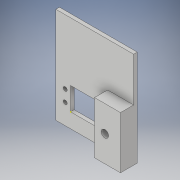
# Autodesk Inventor part: ClawServoHolder
Saved by Autodesk Inventor 2017 (Build 210142000, 142)
## iProperties
Created: 2017-09-23
Part Number: ClawServoHolder
Material: Generic
Document SubType Name: Modeling
Designer: User
Density: 1 g/cm^3
Appearance: Default
Author: User
Autodesk Inventor part; units mm, degrees
ref_plane "YZ Plane" through (0, 0, 0) normal (1, 0, 0) x (0, 1, 0)
ref_plane "XZ Plane" through (0, 0, 0) normal (0, 1, 0) x (-1, 0, 0)
ref_plane "XY Plane" through (0, 0, 0) normal (0, 0, 1) x (1, 0, 0)
sketch "Sketch1" plane through (0, 0, 0) normal (0, 0, 1) x (1, 0, 0)
  line L0 (0, 0) -> (38.8112, 0)
  line L1 (38.8112, 0) -> (38.8112, 19.812)
  line L2 (38.8112, 19.812) -> (0, 19.812)
  line L3 (0, 19.812) -> (0, 0)
  line L4 (-12.7, -12.7) -> (-12.7, 32.512)
  line L5 (-12.7, 32.512) -> (51.5112, 32.512)
  line L6 (51.5112, 32.512) -> (51.5112, -12.7)
  line L7 (-12.7, -12.7) -> (51.5112, -12.7)
  dimension "d0" = 38.8112
  dimension "d1" = 19.812
  constraints: 16 end point, 3 perpendicular, 2 horizontal, 2 parallel
  measures "d0" distance of L2.end L1.end
  measures "d1" distance of L1.end L0.end
extrude "Extrusion1" add sketch "Sketch1" along normal blind 3.175
sketch "Sketch2" plane through (0, 0, 3.175) normal (0, 0, 1) x (1, 0, 0)
  line L0 (0, 19.812) -> (0, 0) projected
  circle A0 centre (-4.5974, 4.9022) radius 1.0541
  line L1 (38.8112, 19.812) -> (38.8112, 0) projected
  circle A1 centre (43.4086, 4.9022) radius 1.0541
  circle A2 centre (43.4086, 14.9098) radius 1.0541
  circle A3 centre (-4.5974, 14.9098) radius 1.0541
  circle A4 centre (-4.5974, 4.9022) radius 1.7145
  circle A5 centre (-4.5974, 14.9098) radius 1.7145
  circle A6 centre (43.4086, 14.9098) radius 1.7145
  circle A7 centre (43.4086, 4.9022) radius 1.7145
  dimension "d10" = 2.1082
  dimension "d15" = 3.429
  dimension "d16" = 3.429
  dimension "d17" = 3.429
  dimension "d18" = 3.429
  dimension "d46" = 48.006
  dimension "d47" = 48.006
  constraints: 8 centre point, 5 coincident
  measures "d10" diameter of A0
  measures "d15" diameter of A4
  measures "d16" diameter of A5
  measures "d17" diameter of A6
  measures "d18" diameter of A7
  measures "d46" distance of A2.centre A3.centre
  measures "d47" distance of A1.centre A0.centre
extrude "Extrusion2" cut sketch "Sketch2" against normal blind 3.175 contours A0 | A1 | A2 | A3 | A4 | A5 | A6 | A7
sketch "Sketch3" plane through (51.5112, -12.7, 0) normal (1, 0, 0) x (0, 0, -1)
  line L0 (0, 0) -> (-3.175, 0) projected
  line L1 (-3.175, 0) -> (-3.175, 45.212) projected
  line L2 (0, 0) -> (-3.175, 0)
  line L3 (-3.175, 0) -> (-3.175, 45.212)
  line L4 (-3.175, 45.212) -> (0, 45.212)
  line L5 (0, 45.212) -> (0, 0)
  point P0 (0, 12.7)
  constraints: 8 end point, 2 parallel, 1 horizontal, 1 perpendicular
extrude "Extrusion3" add sketch "Sketch3" along normal blind 3.175
sketch "Sketch4" plane through (0, 0, 3.175) normal (0, 0, 1) x (1, 0, 0)
  line L0 (54.6862, 32.512) -> (54.6862, -12.7) projected
  line L1 (54.6862, 32.512) -> (51.5112, 32.512)
  line L2 (-12.7, 32.512) -> (54.6862, 32.512) projected
  line L3 (51.5112, 32.512) -> (51.2299, -12.7)
  line L4 (-12.7, -12.7) -> (54.6862, -12.7) projected
  line L5 (54.6862, -12.7) -> (51.2299, -12.7)
  point P0 (0, 0)
  dimension "d21" = 3.175
  constraints: 6 end point, 2 point on line, 1 collinear
  measures "d21" distance of L0.start L1.end
extrude "Extrusion4" add sketch "Sketch4" along normal blind 8.2296
sketch "Sketch8" plane through (0, 0, 3.175) normal (0, 0, 1) x (1, 0, 0)
  line L0 (51.2299, -12.7) -> (32.1799, -12.7)
  line L1 (-12.7, -12.7) -> (51.2299, -12.7) projected
  line L2 (38.8112, 0) -> (0, 0) projected
  line L3 (32.1799, -12.7) -> (32.1799, 32.512)
  line L4 (-12.7, 32.512) -> (51.5112, 32.512) projected
  line L5 (32.1799, 32.512) -> (51.5112, 32.512)
  line L6 (51.2299, -12.7) -> (51.5112, 32.512) projected
  line L7 (51.5112, 32.512) -> (51.2299, -12.7)
  dimension "d33" = 19.05
  dimension "d36" = 45.212
  constraints: 8 end point, 2 collinear, 2 point on line
  measures "d33" distance of L0.start L0.end
  measures "d36" distance of L0.end L3.end
extrude "Extrusion7" add sketch "Sketch8" along normal blind 8.2296
sketch "Sketch9" plane through (0, 0, 11.4046) normal (0, 0, 1) x (1, 0, 0)
  line L0 (54.6862, -12.7) -> (54.6862, 32.512) projected
  line L1 (54.6862, 8.6893) -> (68.1482, 8.6893) construction
  line L2 (-12.7, 32.512) -> (54.6862, 32.512) projected
  line L3 (41.2242, 32.512) -> (63.8302, 32.512) construction
  circle A0 centre (41.2242, 9.906) radius 3.175
  point P0 (0, 0)
  dimension "d41" = 6.35
  constraints: 4 end point, 2 horizontal, 2 point on line, 1 centre point
  measures "d41" diameter of A0
sketch "Sketch10" plane through (0, 0, 3.175) normal (0, 0, -1) x (-1, 0, 0)
  line L0 (-38.8112, 0) -> (-38.8112, 19.812) projected
  line L1 (-38.8112, 19.812) -> (-38.8112, 0)
  line L2 (-38.8112, 0) -> (-32.1799, 0)
  line L3 (-32.1799, 32.512) -> (-32.1799, -12.7) projected
  line L4 (-32.1799, 19.812) -> (-32.1799, 0)
  line L5 (-38.8112, 19.812) -> (0, 19.812) projected
  line L6 (-38.8112, 19.812) -> (-32.1799, 19.812)
  point P0 (0, 0)
  constraints: 8 end point, 3 collinear, 2 point on line, 1 perpendicular
extrude "Extrusion9" cut sketch "Sketch10" against normal blind 5.08
thread "Thread1" size "6-32 UNC" class "2B" standard "ANSI Unified Screw Threads" full length
thread "Thread2" size "6-32 UNC" class "2B" standard "ANSI Unified Screw Threads" full length
thread "Thread3" size "6-32 UNC" class "2B" standard "ANSI Unified Screw Threads" full length
thread "Thread4" size "6-32 UNC" class "2B" standard "ANSI Unified Screw Threads" full length
sketch "Sketch11" plane through (0, 0, 11.4046) normal (0, 0, 1) x (1, 0, 0)
  line L0 (54.6862, 32.512) -> (32.1799, 32.512) projected
  line L1 (54.6862, -12.7) -> (32.1799, -12.7)
  line L2 (32.1799, -12.7) -> (32.1799, 32.512)
  line L3 (32.1799, 32.512) -> (54.6862, 32.512)
  line L4 (54.6862, 32.512) -> (54.6862, -12.7)
  point P0 (0, 0)
  constraints: 8 end point, 2 parallel, 1 horizontal, 1 perpendicular
extrude "Extrusion10" add sketch "Sketch11" along normal blind 3.175
sketch "Sketch12" plane through (0, 0, 14.5796) normal (0, 0, 1) x (1, 0, 0)
  line L0 (32.1799, 32.512) -> (32.1799, -12.7) projected
  line L1 (32.1799, 9.906) -> (41.2223, 9.906)
  circle A0 centre (41.2223, 9.906) radius 3.175
  circle A1 centre (43.4086, 4.9022) radius 1.7145 projected
  line L2 (32.1799, -12.7) -> (54.6862, -12.7) projected
  line L3 (54.6862, -12.7) -> (54.6862, 32.512) projected
  line L4 (54.6862, 32.512) -> (32.1799, 32.512) projected
  line L5 (32.1799, 32.512) -> (32.1799, -12.7) projected
  line L6 (32.1799, -12.7) -> (54.6862, -12.7) projected
  line L7 (54.6862, -12.7) -> (54.6862, 32.512) projected
  line L8 (54.6862, 32.512) -> (32.1799, 32.512) projected
  line L9 (32.1799, 32.512) -> (32.1799, -12.7) projected
  line L10 (32.1799, -12.7) -> (54.6862, -12.7) projected
  line L11 (54.6862, -12.7) -> (54.6862, 32.512) projected
  line L12 (54.6862, 32.512) -> (32.1799, 32.512) projected
  line L13 (32.1799, 32.512) -> (32.1799, -12.7) projected
  point P0 (0, 0)
  dimension "d58" = 9.0424
  dimension "d59" = 6.35
  constraints: 2 end point, 1 centre point, 1 coincident, 1 horizontal, 1 midpoint
  measures "d58" distance of L1.start L1.end
  measures "d59" diameter of A0
hole "Hole1" at (41.2223, 9.906, 14.5796) direction (0, 0, -1) diameter 6.35 depth 6.35
sketch "Sketch13" plane through (0, 0, 8.255) normal (0, 0, -1) x (-1, 0, 0)
  line L0 (-38.8112, 0) -> (-38.8112, 19.812) projected
  line L1 (-38.8112, 19.812) -> (-32.1799, 19.812) projected
  line L2 (-38.8112, 0) -> (-32.1799, 0)
  line L3 (-32.1799, 0) -> (-32.1799, 19.812)
  line L4 (-32.1799, 19.812) -> (-38.8112, 19.812)
  line L5 (-38.8112, 19.812) -> (-38.8112, 0)
  point P0 (0, 0)
  constraints: 8 end point, 2 parallel, 1 horizontal, 1 perpendicular
extrude "Extrusion11" add sketch "Sketch13" along normal blind 0.254
sketch "Sketch14" plane through (0, 0, 3.175) normal (0, 0, 1) x (1, 0, 0)
  point P0 (0, 0)
sketch "Sketch15" plane through (-12.7, 32.512, 3.175) normal (0, 1, 0) x (1, 0, 0)
  line L0 (67.3862, 3.175) -> (67.3862, -11.4046) projected
  line L1 (0, 0) -> (67.3862, 0)
  line L2 (67.3862, 0) -> (67.3862, 3.175)
  line L3 (67.3862, 3.175) -> (0, 3.175)
  line L4 (0, 3.175) -> (0, 0)
  point P0 (12.7, 3.175)
  constraints: 8 end point, 2 parallel, 1 horizontal, 1 perpendicular
extrude "Extrusion12" add sketch "Sketch15" along normal blind 38.1
body "Solid1"
